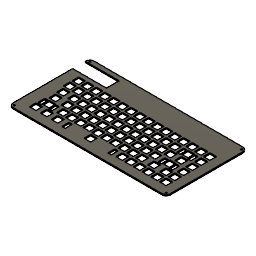
middle (Autodesk Fusion 360 design; units mm, degrees)
part number: 2026-05-16-15-46-12-709
Autodesk Fusion 360 part; units mm, degrees
(part 1 of 3)
sketch "Sketch1" plane through (0, 0, 0) normal (0, 0, 1) x (1, 0, 0)
  line L0 (228.9474, 57.4273) -> (228.9474, -118.8427)
  line L1 (-113.7226, 57.4273) -> (228.9474, 57.4273)
  line L2 (-113.7226, -118.8427) -> (-113.7226, 57.4273)
  line L3 (228.9474, -118.8427) -> (-113.7226, -118.8427)
  line L4 (-90.3928, 10.2823) -> (-77.3928, 10.2823)
  line L5 (-90.3928, -3.7177) -> (-77.3928, -3.7177)
  line L6 (-90.8928, 9.7823) -> (-90.8928, -3.2177)
  line L7 (-76.8928, 9.7823) -> (-76.8928, -3.2177)
  arc A0 (-90.3928, 10.2823) -> (-90.8928, 9.7823) centre (-90.3928, 9.7823) ccw
  arc A1 (-76.8928, 9.7823) -> (-77.3928, 10.2823) centre (-77.3928, 9.7823) ccw
  arc A2 (-90.8928, -3.2177) -> (-90.3928, -3.7177) centre (-90.3928, -3.2177) ccw
  arc A3 (-77.3928, -3.7177) -> (-76.8928, -3.2177) centre (-77.3928, -3.2177) ccw
  line L8 (-71.3428, 10.2823) -> (-58.3428, 10.2823)
  line L9 (-71.3428, -3.7177) -> (-58.3428, -3.7177)
  line L10 (-71.8428, 9.7823) -> (-71.8428, -3.2177)
  line L11 (-57.8428, 9.7823) -> (-57.8428, -3.2177)
  arc A4 (-71.3428, 10.2823) -> (-71.8428, 9.7823) centre (-71.3428, 9.7823) ccw
  arc A5 (-57.8428, 9.7823) -> (-58.3428, 10.2823) centre (-58.3428, 9.7823) ccw
  arc A6 (-71.8428, -3.2177) -> (-71.3428, -3.7177) centre (-71.3428, -3.2177) ccw
  arc A7 (-58.3428, -3.7177) -> (-57.8428, -3.2177) centre (-58.3428, -3.2177) ccw
  line L12 (-52.2928, 10.2823) -> (-39.2928, 10.2823)
  line L13 (-52.2928, -3.7177) -> (-39.2928, -3.7177)
  line L14 (-52.7928, 9.7823) -> (-52.7928, -3.2177)
  line L15 (-38.7928, 9.7823) -> (-38.7928, -3.2177)
  arc A8 (-52.2928, 10.2823) -> (-52.7928, 9.7823) centre (-52.2928, 9.7823) ccw
  arc A9 (-38.7928, 9.7823) -> (-39.2928, 10.2823) centre (-39.2928, 9.7823) ccw
  arc A10 (-52.7928, -3.2177) -> (-52.2928, -3.7177) centre (-52.2928, -3.2177) ccw
  arc A11 (-39.2928, -3.7177) -> (-38.7928, -3.2177) centre (-39.2928, -3.2177) ccw
  line L16 (-33.2428, 10.2823) -> (-20.2428, 10.2823)
  line L17 (-33.2428, -3.7177) -> (-20.2428, -3.7177)
  line L18 (-33.7428, 9.7823) -> (-33.7428, -3.2177)
  line L19 (-19.7428, 9.7823) -> (-19.7428, -3.2177)
  arc A12 (-33.2428, 10.2823) -> (-33.7428, 9.7823) centre (-33.2428, 9.7823) ccw
  arc A13 (-19.7428, 9.7823) -> (-20.2428, 10.2823) centre (-20.2428, 9.7823) ccw
  arc A14 (-33.7428, -3.2177) -> (-33.2428, -3.7177) centre (-33.2428, -3.2177) ccw
  arc A15 (-20.2428, -3.7177) -> (-19.7428, -3.2177) centre (-20.2428, -3.2177) ccw
  line L20 (-14.1928, 10.2823) -> (-1.1928, 10.2823)
  line L21 (-14.1928, -3.7177) -> (-1.1928, -3.7177)
  line L22 (-14.6928, 9.7823) -> (-14.6928, -3.2177)
  line L23 (-0.6928, 9.7823) -> (-0.6928, -3.2177)
  arc A16 (-14.1928, 10.2823) -> (-14.6928, 9.7823) centre (-14.1928, 9.7823) ccw
  arc A17 (-0.6928, 9.7823) -> (-1.1928, 10.2823) centre (-1.1928, 9.7823) ccw
  arc A18 (-14.6928, -3.2177) -> (-14.1928, -3.7177) centre (-14.1928, -3.2177) ccw
  arc A19 (-1.1928, -3.7177) -> (-0.6928, -3.2177) centre (-1.1928, -3.2177) ccw
  line L24 (4.8572, 10.2823) -> (17.8572, 10.2823)
  line L25 (4.8572, -3.7177) -> (17.8572, -3.7177)
  line L26 (4.3572, 9.7823) -> (4.3572, -3.2177)
  line L27 (18.3572, 9.7823) -> (18.3572, -3.2177)
  arc A20 (4.8572, 10.2823) -> (4.3572, 9.7823) centre (4.8572, 9.7823) ccw
  arc A21 (18.3572, 9.7823) -> (17.8572, 10.2823) centre (17.8572, 9.7823) ccw
  arc A22 (4.3572, -3.2177) -> (4.8572, -3.7177) centre (4.8572, -3.2177) ccw
  arc A23 (17.8572, -3.7177) -> (18.3572, -3.2177) centre (17.8572, -3.2177) ccw
  line L28 (23.9072, 10.2823) -> (36.9072, 10.2823)
  line L29 (23.9072, -3.7177) -> (36.9072, -3.7177)
  line L30 (23.4072, 9.7823) -> (23.4072, -3.2177)
  line L31 (37.4072, 9.7823) -> (37.4072, -3.2177)
  arc A24 (23.9072, 10.2823) -> (23.4072, 9.7823) centre (23.9072, 9.7823) ccw
  arc A25 (37.4072, 9.7823) -> (36.9072, 10.2823) centre (36.9072, 9.7823) ccw
  arc A26 (23.4072, -3.2177) -> (23.9072, -3.7177) centre (23.9072, -3.2177) ccw
  arc A27 (36.9072, -3.7177) -> (37.4072, -3.2177) centre (36.9072, -3.2177) ccw
  line L32 (42.9572, 10.2823) -> (55.9572, 10.2823)
  line L33 (42.9572, -3.7177) -> (55.9572, -3.7177)
  line L34 (42.4572, 9.7823) -> (42.4572, -3.2177)
  line L35 (56.4572, 9.7823) -> (56.4572, -3.2177)
  arc A28 (42.9572, 10.2823) -> (42.4572, 9.7823) centre (42.9572, 9.7823) ccw
  arc A29 (56.4572, 9.7823) -> (55.9572, 10.2823) centre (55.9572, 9.7823) ccw
  arc A30 (42.4572, -3.2177) -> (42.9572, -3.7177) centre (42.9572, -3.2177) ccw
  arc A31 (55.9572, -3.7177) -> (56.4572, -3.2177) centre (55.9572, -3.2177) ccw
  line L36 (62.0072, 10.2823) -> (75.0072, 10.2823)
  line L37 (62.0072, -3.7177) -> (75.0072, -3.7177)
  line L38 (61.5072, 9.7823) -> (61.5072, -3.2177)
  line L39 (75.5072, 9.7823) -> (75.5072, -3.2177)
  arc A32 (62.0072, 10.2823) -> (61.5072, 9.7823) centre (62.0072, 9.7823) ccw
  arc A33 (75.5072, 9.7823) -> (75.0072, 10.2823) centre (75.0072, 9.7823) ccw
  arc A34 (61.5072, -3.2177) -> (62.0072, -3.7177) centre (62.0072, -3.2177) ccw
  arc A35 (75.0072, -3.7177) -> (75.5072, -3.2177) centre (75.0072, -3.2177) ccw
  line L40 (81.0572, 10.2823) -> (94.0572, 10.2823)
  line L41 (81.0572, -3.7177) -> (94.0572, -3.7177)
  line L42 (80.5572, 9.7823) -> (80.5572, -3.2177)
  line L43 (94.5572, 9.7823) -> (94.5572, -3.2177)
  arc A36 (81.0572, 10.2823) -> (80.5572, 9.7823) centre (81.0572, 9.7823) ccw
  arc A37 (94.5572, 9.7823) -> (94.0572, 10.2823) centre (94.0572, 9.7823) ccw
  arc A38 (80.5572, -3.2177) -> (81.0572, -3.7177) centre (81.0572, -3.2177) ccw
  arc A39 (94.0572, -3.7177) -> (94.5572, -3.2177) centre (94.0572, -3.2177) ccw
  line L44 (100.1072, 10.2823) -> (113.1072, 10.2823)
  line L45 (100.1072, -3.7177) -> (113.1072, -3.7177)
  line L46 (99.6072, 9.7823) -> (99.6072, -3.2177)
  line L47 (113.6072, 9.7823) -> (113.6072, -3.2177)
  arc A40 (100.1072, 10.2823) -> (99.6072, 9.7823) centre (100.1072, 9.7823) ccw
  arc A41 (113.6072, 9.7823) -> (113.1072, 10.2823) centre (113.1072, 9.7823) ccw
  arc A42 (99.6072, -3.2177) -> (100.1072, -3.7177) centre (100.1072, -3.2177) ccw
  arc A43 (113.1072, -3.7177) -> (113.6072, -3.2177) centre (113.1072, -3.2177) ccw
  line L48 (119.1572, 10.2823) -> (132.1572, 10.2823)
  line L49 (119.1572, -3.7177) -> (132.1572, -3.7177)
  line L50 (118.6572, 9.7823) -> (118.6572, -3.2177)
  line L51 (132.6572, 9.7823) -> (132.6572, -3.2177)
  arc A44 (119.1572, 10.2823) -> (118.6572, 9.7823) centre (119.1572, 9.7823) ccw
  arc A45 (132.6572, 9.7823) -> (132.1572, 10.2823) centre (132.1572, 9.7823) ccw
  arc A46 (118.6572, -3.2177) -> (119.1572, -3.7177) centre (119.1572, -3.2177) ccw
  arc A47 (132.1572, -3.7177) -> (132.6572, -3.2177) centre (132.1572, -3.2177) ccw
  line L52 (138.2072, 10.2823) -> (151.2072, 10.2823)
  line L53 (138.2072, -3.7177) -> (151.2072, -3.7177)
  line L54 (137.7072, 9.7823) -> (137.7072, -3.2177)
  line L55 (151.7072, 9.7823) -> (151.7072, -3.2177)
  arc A48 (138.2072, 10.2823) -> (137.7072, 9.7823) centre (138.2072, 9.7823) ccw
  arc A49 (151.7072, 9.7823) -> (151.2072, 10.2823) centre (151.2072, 9.7823) ccw
  arc A50 (137.7072, -3.2177) -> (138.2072, -3.7177) centre (138.2072, -3.2177) ccw
  arc A51 (151.2072, -3.7177) -> (151.7072, -3.2177) centre (151.2072, -3.2177) ccw
  line L56 (157.2572, 10.2823) -> (170.2572, 10.2823)
  line L57 (157.2572, -3.7177) -> (170.2572, -3.7177)
  line L58 (156.7572, 9.7823) -> (156.7572, -3.2177)
  line L59 (170.7572, 9.7823) -> (170.7572, -3.2177)
  arc A52 (157.2572, 10.2823) -> (156.7572, 9.7823) centre (157.2572, 9.7823) ccw
  arc A53 (170.7572, 9.7823) -> (170.2572, 10.2823) centre (170.2572, 9.7823) ccw
  arc A54 (156.7572, -3.2177) -> (157.2572, -3.7177) centre (157.2572, -3.2177) ccw
  arc A55 (170.2572, -3.7177) -> (170.7572, -3.2177) centre (170.2572, -3.2177) ccw
  line L60 (176.3072, 10.2823) -> (189.3072, 10.2823)
  line L61 (176.3072, -3.7177) -> (189.3072, -3.7177)
  line L62 (175.8072, 9.7823) -> (175.8072, -3.2177)
  line L63 (189.8072, 9.7823) -> (189.8072, -3.2177)
  arc A56 (176.3072, 10.2823) -> (175.8072, 9.7823) centre (176.3072, 9.7823) ccw
  arc A57 (189.8072, 9.7823) -> (189.3072, 10.2823) centre (189.3072, 9.7823) ccw
  arc A58 (175.8072, -3.2177) -> (176.3072, -3.7177) centre (176.3072, -3.2177) ccw
  arc A59 (189.3072, -3.7177) -> (189.8072, -3.2177) centre (189.3072, -3.2177) ccw
  line L64 (195.3572, 10.2823) -> (208.3572, 10.2823)
  line L65 (195.3572, -3.7177) -> (208.3572, -3.7177)
  line L66 (194.8572, 9.7823) -> (194.8572, -3.2177)
  line L67 (208.8572, 9.7823) -> (208.8572, -3.2177)
  arc A60 (195.3572, 10.2823) -> (194.8572, 9.7823) centre (195.3572, 9.7823) ccw
  arc A61 (208.8572, 9.7823) -> (208.3572, 10.2823) centre (208.3572, 9.7823) ccw
  arc A62 (194.8572, -3.2177) -> (195.3572, -3.7177) centre (195.3572, -3.2177) ccw
  arc A63 (208.3572, -3.7177) -> (208.8572, -3.2177) centre (208.3572, -3.2177) ccw
  line L68 (-90.3928, -8.7677) -> (-77.3928, -8.7677)
  line L69 (-90.3928, -22.7677) -> (-77.3928, -22.7677)
  line L70 (-90.8928, -9.2677) -> (-90.8928, -22.2677)
  line L71 (-76.8928, -9.2677) -> (-76.8928, -22.2677)
  arc A64 (-90.3928, -8.7677) -> (-90.8928, -9.2677) centre (-90.3928, -9.2677) ccw
  arc A65 (-76.8928, -9.2677) -> (-77.3928, -8.7677) centre (-77.3928, -9.2677) ccw
  arc A66 (-90.8928, -22.2677) -> (-90.3928, -22.7677) centre (-90.3928, -22.2677) ccw
  arc A67 (-77.3928, -22.7677) -> (-76.8928, -22.2677) centre (-77.3928, -22.2677) ccw
  line L72 (-71.3428, -8.7677) -> (-58.3428, -8.7677)
  line L73 (-71.3428, -22.7677) -> (-58.3428, -22.7677)
  line L74 (-71.8428, -9.2677) -> (-71.8428, -22.2677)
  line L75 (-57.8428, -9.2677) -> (-57.8428, -22.2677)
  arc A68 (-71.3428, -8.7677) -> (-71.8428, -9.2677) centre (-71.3428, -9.2677) ccw
  arc A69 (-57.8428, -9.2677) -> (-58.3428, -8.7677) centre (-58.3428, -9.2677) ccw
  arc A70 (-71.8428, -22.2677) -> (-71.3428, -22.7677) centre (-71.3428, -22.2677) ccw
  arc A71 (-58.3428, -22.7677) -> (-57.8428, -22.2677) centre (-58.3428, -22.2677) ccw
  line L76 (-52.2928, -8.7677) -> (-39.2928, -8.7677)
  line L77 (-52.2928, -22.7677) -> (-39.2928, -22.7677)
  line L78 (-52.7928, -9.2677) -> (-52.7928, -22.2677)
  line L79 (-38.7928, -9.2677) -> (-38.7928, -22.2677)
  arc A72 (-52.2928, -8.7677) -> (-52.7928, -9.2677) centre (-52.2928, -9.2677) ccw
  arc A73 (-38.7928, -9.2677) -> (-39.2928, -8.7677) centre (-39.2928, -9.2677) ccw
  arc A74 (-52.7928, -22.2677) -> (-52.2928, -22.7677) centre (-52.2928, -22.2677) ccw
  arc A75 (-39.2928, -22.7677) -> (-38.7928, -22.2677) centre (-39.2928, -22.2677) ccw
  line L80 (-33.2428, -8.7677) -> (-20.2428, -8.7677)
  line L81 (-33.2428, -22.7677) -> (-20.2428, -22.7677)
  line L82 (-33.7428, -9.2677) -> (-33.7428, -22.2677)
  line L83 (-19.7428, -9.2677) -> (-19.7428, -22.2677)
  arc A76 (-33.2428, -8.7677) -> (-33.7428, -9.2677) centre (-33.2428, -9.2677) ccw
  arc A77 (-19.7428, -9.2677) -> (-20.2428, -8.7677) centre (-20.2428, -9.2677) ccw
  arc A78 (-33.7428, -22.2677) -> (-33.2428, -22.7677) centre (-33.2428, -22.2677) ccw
  arc A79 (-20.2428, -22.7677) -> (-19.7428, -22.2677) centre (-20.2428, -22.2677) ccw
  line L84 (-14.1928, -8.7677) -> (-1.1928, -8.7677)
  line L85 (-14.1928, -22.7677) -> (-1.1928, -22.7677)
  line L86 (-14.6928, -9.2677) -> (-14.6928, -22.2677)
  line L87 (-0.6928, -9.2677) -> (-0.6928, -22.2677)
  arc A80 (-14.1928, -8.7677) -> (-14.6928, -9.2677) centre (-14.1928, -9.2677) ccw
  arc A81 (-0.6928, -9.2677) -> (-1.1928, -8.7677) centre (-1.1928, -9.2677) ccw
  arc A82 (-14.6928, -22.2677) -> (-14.1928, -22.7677) centre (-14.1928, -22.2677) ccw
  arc A83 (-1.1928, -22.7677) -> (-0.6928, -22.2677) centre (-1.1928, -22.2677) ccw
  line L88 (4.8572, -8.7677) -> (17.8572, -8.7677)
  line L89 (4.8572, -22.7677) -> (17.8572, -22.7677)
  line L90 (4.3572, -9.2677) -> (4.3572, -22.2677)
  line L91 (18.3572, -9.2677) -> (18.3572, -22.2677)
  arc A84 (4.8572, -8.7677) -> (4.3572, -9.2677) centre (4.8572, -9.2677) ccw
  arc A85 (18.3572, -9.2677) -> (17.8572, -8.7677) centre (17.8572, -9.2677) ccw
  arc A86 (4.3572, -22.2677) -> (4.8572, -22.7677) centre (4.8572, -22.2677) ccw
  arc A87 (17.8572, -22.7677) -> (18.3572, -22.2677) centre (17.8572, -22.2677) ccw
  line L92 (23.9072, -8.7677) -> (36.9072, -8.7677)
  line L93 (23.9072, -22.7677) -> (36.9072, -22.7677)
  line L94 (23.4072, -9.2677) -> (23.4072, -22.2677)
  line L95 (37.4072, -9.2677) -> (37.4072, -22.2677)
  arc A88 (23.9072, -8.7677) -> (23.4072, -9.2677) centre (23.9072, -9.2677) ccw
  arc A89 (37.4072, -9.2677) -> (36.9072, -8.7677) centre (36.9072, -9.2677) ccw
  arc A90 (23.4072, -22.2677) -> (23.9072, -22.7677) centre (23.9072, -22.2677) ccw
  arc A91 (36.9072, -22.7677) -> (37.4072, -22.2677) centre (36.9072, -22.2677) ccw
  line L96 (42.9572, -8.7677) -> (55.9572, -8.7677)
  line L97 (42.9572, -22.7677) -> (55.9572, -22.7677)
  line L98 (42.4572, -9.2677) -> (42.4572, -22.2677)
  line L99 (56.4572, -9.2677) -> (56.4572, -22.2677)
  arc A92 (42.9572, -8.7677) -> (42.4572, -9.2677) centre (42.9572, -9.2677) ccw
  arc A93 (56.4572, -9.2677) -> (55.9572, -8.7677) centre (55.9572, -9.2677) ccw
  arc A94 (42.4572, -22.2677) -> (42.9572, -22.7677) centre (42.9572, -22.2677) ccw
  arc A95 (55.9572, -22.7677) -> (56.4572, -22.2677) centre (55.9572, -22.2677) ccw
  line L100 (62.0072, -8.7677) -> (75.0072, -8.7677)
  line L101 (62.0072, -22.7677) -> (75.0072, -22.7677)
  line L102 (61.5072, -9.2677) -> (61.5072, -22.2677)
  line L103 (75.5072, -9.2677) -> (75.5072, -22.2677)
  arc A96 (62.0072, -8.7677) -> (61.5072, -9.2677) centre (62.0072, -9.2677) ccw
  arc A97 (75.5072, -9.2677) -> (75.0072, -8.7677) centre (75.0072, -9.2677) ccw
  arc A98 (61.5072, -22.2677) -> (62.0072, -22.7677) centre (62.0072, -22.2677) ccw
  arc A99 (75.0072, -22.7677) -> (75.5072, -22.2677) centre (75.0072, -22.2677) ccw
  line L104 (81.0572, -8.7677) -> (94.0572, -8.7677)
  line L105 (81.0572, -22.7677) -> (94.0572, -22.7677)
  line L106 (80.5572, -9.2677) -> (80.5572, -22.2677)
  line L107 (94.5572, -9.2677) -> (94.5572, -22.2677)
  arc A100 (81.0572, -8.7677) -> (80.5572, -9.2677) centre (81.0572, -9.2677) ccw
  arc A101 (94.5572, -9.2677) -> (94.0572, -8.7677) centre (94.0572, -9.2677) ccw
  arc A102 (80.5572, -22.2677) -> (81.0572, -22.7677) centre (81.0572, -22.2677) ccw
  arc A103 (94.0572, -22.7677) -> (94.5572, -22.2677) centre (94.0572, -22.2677) ccw
  line L108 (100.1072, -8.7677) -> (113.1072, -8.7677)
  line L109 (100.1072, -22.7677) -> (113.1072, -22.7677)
  line L110 (99.6072, -9.2677) -> (99.6072, -22.2677)
  line L111 (113.6072, -9.2677) -> (113.6072, -22.2677)
  arc A104 (100.1072, -8.7677) -> (99.6072, -9.2677) centre (100.1072, -9.2677) ccw
  arc A105 (113.6072, -9.2677) -> (113.1072, -8.7677) centre (113.1072, -9.2677) ccw
  arc A106 (99.6072, -22.2677) -> (100.1072, -22.7677) centre (100.1072, -22.2677) ccw
  arc A107 (113.1072, -22.7677) -> (113.6072, -22.2677) centre (113.1072, -22.2677) ccw
  line L112 (119.1572, -8.7677) -> (132.1572, -8.7677)
  line L113 (119.1572, -22.7677) -> (132.1572, -22.7677)
  line L114 (118.6572, -9.2677) -> (118.6572, -22.2677)
  line L115 (132.6572, -9.2677) -> (132.6572, -22.2677)
  arc A108 (119.1572, -8.7677) -> (118.6572, -9.2677) centre (119.1572, -9.2677) ccw
  arc A109 (132.6572, -9.2677) -> (132.1572, -8.7677) centre (132.1572, -9.2677) ccw
  arc A110 (118.6572, -22.2677) -> (119.1572, -22.7677) centre (119.1572, -22.2677) ccw
  arc A111 (132.1572, -22.7677) -> (132.6572, -22.2677) centre (132.1572, -22.2677) ccw
  line L116 (138.2072, -8.7677) -> (151.2072, -8.7677)
  line L117 (138.2072, -22.7677) -> (151.2072, -22.7677)
  line L118 (137.7072, -9.2677) -> (137.7072, -22.2677)
  line L119 (151.7072, -9.2677) -> (151.7072, -22.2677)
  arc A112 (138.2072, -8.7677) -> (137.7072, -9.2677) centre (138.2072, -9.2677) ccw
  arc A113 (151.7072, -9.2677) -> (151.2072, -8.7677) centre (151.2072, -9.2677) ccw
  arc A114 (137.7072, -22.2677) -> (138.2072, -22.7677) centre (138.2072, -22.2677) ccw
  arc A115 (151.2072, -22.7677) -> (151.7072, -22.2677) centre (151.2072, -22.2677) ccw
  line L120 (166.7822, -8.7677) -> (179.7822, -8.7677)
  line L121 (166.7822, -22.7677) -> (179.7822, -22.7677)
  line L122 (166.2822, -9.2677) -> (166.2822, -22.2677)
  line L123 (180.2822, -9.2677) -> (180.2822, -22.2677)
  arc A116 (166.7822, -8.7677) -> (166.2822, -9.2677) centre (166.7822, -9.2677) ccw
  arc A117 (180.2822, -9.2677) -> (179.7822, -8.7677) centre (179.7822, -9.2677) ccw
  arc A118 (166.2822, -22.2677) -> (166.7822, -22.7677) centre (166.7822, -22.2677) ccw
  arc A119 (179.7822, -22.7677) -> (180.2822, -22.2677) centre (179.7822, -22.2677) ccw
  line L124 (158.3442, -9.7677) -> (164.3442, -9.7677)
  line L125 (158.3442, -24.7677) -> (164.3442, -24.7677)
  line L126 (157.8442, -10.2677) -> (157.8442, -24.2677)
  line L127 (164.8442, -10.2677) -> (164.8442, -24.2677)
  arc A120 (158.3442, -9.7677) -> (157.8442, -10.2677) centre (158.3442, -10.2677) ccw
  arc A121 (164.8442, -10.2677) -> (164.3442, -9.7677) centre (164.3442, -10.2677) ccw
  arc A122 (157.8442, -24.2677) -> (158.3442, -24.7677) centre (158.3442, -24.2677) ccw
  arc A123 (164.3442, -24.7677) -> (164.8442, -24.2677) centre (164.3442, -24.2677) ccw
  line L128 (182.2202, -9.7677) -> (188.2202, -9.7677)
  line L129 (182.2202, -24.7677) -> (188.2202, -24.7677)
  line L130 (181.7202, -10.2677) -> (181.7202, -24.2677)
  line L131 (188.7202, -10.2677) -> (188.7202, -24.2677)
  arc A124 (182.2202, -9.7677) -> (181.7202, -10.2677) centre (182.2202, -10.2677) ccw
  arc A125 (188.7202, -10.2677) -> (188.2202, -9.7677) centre (188.2202, -10.2677) ccw
  arc A126 (181.7202, -24.2677) -> (182.2202, -24.7677) centre (182.2202, -24.2677) ccw
  arc A127 (188.2202, -24.7677) -> (188.7202, -24.2677) centre (188.2202, -24.2677) ccw
  line L132 (195.3572, -8.7677) -> (208.3572, -8.7677)
  line L133 (195.3572, -22.7677) -> (208.3572, -22.7677)
  line L134 (194.8572, -9.2677) -> (194.8572, -22.2677)
  line L135 (208.8572, -9.2677) -> (208.8572, -22.2677)
  arc A128 (195.3572, -8.7677) -> (194.8572, -9.2677) centre (195.3572, -9.2677) ccw
  arc A129 (208.8572, -9.2677) -> (208.3572, -8.7677) centre (208.3572, -9.2677) ccw
  arc A130 (194.8572, -22.2677) -> (195.3572, -22.7677) centre (195.3572, -22.2677) ccw
  arc A131 (208.3572, -22.7677) -> (208.8572, -22.2677) centre (208.3572, -22.2677) ccw
  line L136 (-85.6303, -27.8177) -> (-72.6303, -27.8177)
  line L137 (-85.6303, -41.8177) -> (-72.6303, -41.8177)
  line L138 (-86.1303, -28.3177) -> (-86.1303, -41.3177)
  line L139 (-72.1303, -28.3177) -> (-72.1303, -41.3177)
  arc A132 (-85.6303, -27.8177) -> (-86.1303, -28.3177) centre (-85.6303, -28.3177) ccw
  arc A133 (-72.1303, -28.3177) -> (-72.6303, -27.8177) centre (-72.6303, -28.3177) ccw
  arc A134 (-86.1303, -41.3177) -> (-85.6303, -41.8177) centre (-85.6303, -41.3177) ccw
  arc A135 (-72.6303, -41.8177) -> (-72.1303, -41.3177) centre (-72.6303, -41.3177) ccw
  line L140 (-61.8178, -27.8177) -> (-48.8178, -27.8177)
  line L141 (-61.8178, -41.8177) -> (-48.8178, -41.8177)
  line L142 (-62.3178, -28.3177) -> (-62.3178, -41.3177)
  line L143 (-48.3178, -28.3177) -> (-48.3178, -41.3177)
  arc A136 (-61.8178, -27.8177) -> (-62.3178, -28.3177) centre (-61.8178, -28.3177) ccw
  arc A137 (-48.3178, -28.3177) -> (-48.8178, -27.8177) centre (-48.8178, -28.3177) ccw
  arc A138 (-62.3178, -41.3177) -> (-61.8178, -41.8177) centre (-61.8178, -41.3177) ccw
  arc A139 (-48.8178, -41.8177) -> (-48.3178, -41.3177) centre (-48.8178, -41.3177) ccw
  line L144 (-42.7678, -27.8177) -> (-29.7678, -27.8177)
  line L145 (-42.7678, -41.8177) -> (-29.7678, -41.8177)
  line L146 (-43.2678, -28.3177) -> (-43.2678, -41.3177)
  line L147 (-29.2678, -28.3177) -> (-29.2678, -41.3177)
  arc A140 (-42.7678, -27.8177) -> (-43.2678, -28.3177) centre (-42.7678, -28.3177) ccw
  arc A141 (-29.2678, -28.3177) -> (-29.7678, -27.8177) centre (-29.7678, -28.3177) ccw
  arc A142 (-43.2678, -41.3177) -> (-42.7678, -41.8177) centre (-42.7678, -41.3177) ccw
  arc A143 (-29.7678, -41.8177) -> (-29.2678, -41.3177) centre (-29.7678, -41.3177) ccw
  line L148 (-23.7178, -27.8177) -> (-10.7178, -27.8177)
  line L149 (-23.7178, -41.8177) -> (-10.7178, -41.8177)
  line L150 (-24.2178, -28.3177) -> (-24.2178, -41.3177)
  line L151 (-10.2178, -28.3177) -> (-10.2178, -41.3177)
  arc A144 (-23.7178, -27.8177) -> (-24.2178, -28.3177) centre (-23.7178, -28.3177) ccw
  arc A145 (-10.2178, -28.3177) -> (-10.7178, -27.8177) centre (-10.7178, -28.3177) ccw
  arc A146 (-24.2178, -41.3177) -> (-23.7178, -41.8177) centre (-23.7178, -41.3177) ccw
  arc A147 (-10.7178, -41.8177) -> (-10.2178, -41.3177) centre (-10.7178, -41.3177) ccw
  line L152 (-4.6678, -27.8177) -> (8.3322, -27.8177)
  line L153 (-4.6678, -41.8177) -> (8.3322, -41.8177)
  line L154 (-5.1678, -28.3177) -> (-5.1678, -41.3177)
  line L155 (8.8322, -28.3177) -> (8.8322, -41.3177)
  arc A148 (-4.6678, -27.8177) -> (-5.1678, -28.3177) centre (-4.6678, -28.3177) ccw
  arc A149 (8.8322, -28.3177) -> (8.3322, -27.8177) centre (8.3322, -28.3177) ccw
  arc A150 (-5.1678, -41.3177) -> (-4.6678, -41.8177) centre (-4.6678, -41.3177) ccw
  arc A151 (8.3322, -41.8177) -> (8.8322, -41.3177) centre (8.3322, -41.3177) ccw
  line L156 (14.3822, -27.8177) -> (27.3822, -27.8177)
  line L157 (14.3822, -41.8177) -> (27.3822, -41.8177)
  line L158 (13.8822, -28.3177) -> (13.8822, -41.3177)
  line L159 (27.8822, -28.3177) -> (27.8822, -41.3177)
  arc A152 (14.3822, -27.8177) -> (13.8822, -28.3177) centre (14.3822, -28.3177) ccw
  arc A153 (27.8822, -28.3177) -> (27.3822, -27.8177) centre (27.3822, -28.3177) ccw
  arc A154 (13.8822, -41.3177) -> (14.3822, -41.8177) centre (14.3822, -41.3177) ccw
  arc A155 (27.3822, -41.8177) -> (27.8822, -41.3177) centre (27.3822, -41.3177) ccw
  line L160 (33.4322, -27.8177) -> (46.4322, -27.8177)
  line L161 (33.4322, -41.8177) -> (46.4322, -41.8177)
  line L162 (32.9322, -28.3177) -> (32.9322, -41.3177)
  line L163 (46.9322, -28.3177) -> (46.9322, -41.3177)
  arc A156 (33.4322, -27.8177) -> (32.9322, -28.3177) centre (33.4322, -28.3177) ccw
  arc A157 (46.9322, -28.3177) -> (46.4322, -27.8177) centre (46.4322, -28.3177) ccw
  arc A158 (32.9322, -41.3177) -> (33.4322, -41.8177) centre (33.4322, -41.3177) ccw
  arc A159 (46.4322, -41.8177) -> (46.9322, -41.3177) centre (46.4322, -41.3177) ccw
  line L164 (52.4822, -27.8177) -> (65.4822, -27.8177)
  line L165 (52.4822, -41.8177) -> (65.4822, -41.8177)
  line L166 (51.9822, -28.3177) -> (51.9822, -41.3177)
  line L167 (65.9822, -28.3177) -> (65.9822, -41.3177)
  arc A160 (52.4822, -27.8177) -> (51.9822, -28.3177) centre (52.4822, -28.3177) ccw
  arc A161 (65.9822, -28.3177) -> (65.4822, -27.8177) centre (65.4822, -28.3177) ccw
  arc A162 (51.9822, -41.3177) -> (52.4822, -41.8177) centre (52.4822, -41.3177) ccw
  arc A163 (65.4822, -41.8177) -> (65.9822, -41.3177) centre (65.4822, -41.3177) ccw
  line L168 (71.5322, -27.8177) -> (84.5322, -27.8177)
  line L169 (71.5322, -41.8177) -> (84.5322, -41.8177)
  line L170 (71.0322, -28.3177) -> (71.0322, -41.3177)
  line L171 (85.0322, -28.3177) -> (85.0322, -41.3177)
  arc A164 (71.5322, -27.8177) -> (71.0322, -28.3177) centre (71.5322, -28.3177) ccw
  arc A165 (85.0322, -28.3177) -> (84.5322, -27.8177) centre (84.5322, -28.3177) ccw
  arc A166 (71.0322, -41.3177) -> (71.5322, -41.8177) centre (71.5322, -41.3177) ccw
  arc A167 (84.5322, -41.8177) -> (85.0322, -41.3177) centre (84.5322, -41.3177) ccw
  line L172 (90.5822, -27.8177) -> (103.5822, -27.8177)
  line L173 (90.5822, -41.8177) -> (103.5822, -41.8177)
  line L174 (90.0822, -28.3177) -> (90.0822, -41.3177)
  line L175 (104.0822, -28.3177) -> (104.0822, -41.3177)
  arc A168 (90.5822, -27.8177) -> (90.0822, -28.3177) centre (90.5822, -28.3177) ccw
  arc A169 (104.0822, -28.3177) -> (103.5822, -27.8177) centre (103.5822, -28.3177) ccw
  arc A170 (90.0822, -41.3177) -> (90.5822, -41.8177) centre (90.5822, -41.3177) ccw
  arc A171 (103.5822, -41.8177) -> (104.0822, -41.3177) centre (103.5822, -41.3177) ccw
  line L176 (109.6322, -27.8177) -> (122.6322, -27.8177)
  line L177 (109.6322, -41.8177) -> (122.6322, -41.8177)
  line L178 (109.1322, -28.3177) -> (109.1322, -41.3177)
  line L179 (123.1322, -28.3177) -> (123.1322, -41.3177)
  arc A172 (109.6322, -27.8177) -> (109.1322, -28.3177) centre (109.6322, -28.3177) ccw
  arc A173 (123.1322, -28.3177) -> (122.6322, -27.8177) centre (122.6322, -28.3177) ccw
  arc A174 (109.1322, -41.3177) -> (109.6322, -41.8177) centre (109.6322, -41.3177) ccw
  arc A175 (122.6322, -41.8177) -> (123.1322, -41.3177) centre (122.6322, -41.3177) ccw
  line L180 (128.6822, -27.8177) -> (141.6822, -27.8177)
  line L181 (128.6822, -41.8177) -> (141.6822, -41.8177)
  line L182 (128.1822, -28.3177) -> (128.1822, -41.3177)
  line L183 (142.1822, -28.3177) -> (142.1822, -41.3177)
  arc A176 (128.6822, -27.8177) -> (128.1822, -28.3177) centre (128.6822, -28.3177) ccw
  arc A177 (142.1822, -28.3177) -> (141.6822, -27.8177) centre (141.6822, -28.3177) ccw
  arc A178 (128.1822, -41.3177) -> (128.6822, -41.8177) centre (128.6822, -41.3177) ccw
  arc A179 (141.6822, -41.8177) -> (142.1822, -41.3177) centre (141.6822, -41.3177) ccw
  line L184 (147.7322, -27.8177) -> (160.7322, -27.8177)
  line L185 (147.7322, -41.8177) -> (160.7322, -41.8177)
  line L186 (147.2322, -28.3177) -> (147.2322, -41.3177)
  line L187 (161.2322, -28.3177) -> (161.2322, -41.3177)
  arc A180 (147.7322, -27.8177) -> (147.2322, -28.3177) centre (147.7322, -28.3177) ccw
  arc A181 (161.2322, -28.3177) -> (160.7322, -27.8177) centre (160.7322, -28.3177) ccw
  arc A182 (147.2322, -41.3177) -> (147.7322, -41.8177) centre (147.7322, -41.3177) ccw
  arc A183 (160.7322, -41.8177) -> (161.2322, -41.3177) centre (160.7322, -41.3177) ccw
  line L188 (171.5447, -27.8177) -> (184.5447, -27.8177)
  line L189 (171.5447, -41.8177) -> (184.5447, -41.8177)
  line L190 (171.0447, -28.3177) -> (171.0447, -41.3177)
  line L191 (185.0447, -28.3177) -> (185.0447, -41.3177)
  arc A184 (171.5447, -27.8177) -> (171.0447, -28.3177) centre (171.5447, -28.3177) ccw
  arc A185 (185.0447, -28.3177) -> (184.5447, -27.8177) centre (184.5447, -28.3177) ccw
  arc A186 (171.0447, -41.3177) -> (171.5447, -41.8177) centre (171.5447, -41.3177) ccw
  arc A187 (184.5447, -41.8177) -> (185.0447, -41.3177) centre (184.5447, -41.3177) ccw
  line L192 (195.3572, -27.8177) -> (208.3572, -27.8177)
  line L193 (195.3572, -41.8177) -> (208.3572, -41.8177)
  line L194 (194.8572, -28.3177) -> (194.8572, -41.3177)
  line L195 (208.8572, -28.3177) -> (208.8572, -41.3177)
  arc A188 (195.3572, -27.8177) -> (194.8572, -28.3177) centre (195.3572, -28.3177) ccw
  arc A189 (208.8572, -28.3177) -> (208.3572, -27.8177) centre (208.3572, -28.3177) ccw
  arc A190 (194.8572, -41.3177) -> (195.3572, -41.8177) centre (195.3572, -41.3177) ccw
  arc A191 (208.3572, -41.8177) -> (208.8572, -41.3177) centre (208.3572, -41.3177) ccw
  line L196 (-83.2491, -46.8677) -> (-70.2491, -46.8677)
  line L197 (-83.2491, -60.8677) -> (-70.2491, -60.8677)
  line L198 (-83.7491, -47.3677) -> (-83.7491, -60.3677)
  line L199 (-69.7491, -47.3677) -> (-69.7491, -60.3677)
  arc A192 (-83.2491, -46.8677) -> (-83.7491, -47.3677) centre (-83.2491, -47.3677) ccw
  arc A193 (-69.7491, -47.3677) -> (-70.2491, -46.8677) centre (-70.2491, -47.3677) ccw
  arc A194 (-83.7491, -60.3677) -> (-83.2491, -60.8677) centre (-83.2491, -60.3677) ccw
  arc A195 (-70.2491, -60.8677) -> (-69.7491, -60.3677) centre (-70.2491, -60.3677) ccw
  line L200 (-57.0553, -46.8677) -> (-44.0553, -46.8677)
  line L201 (-57.0553, -60.8677) -> (-44.0553, -60.8677)
  line L202 (-57.5553, -47.3677) -> (-57.5553, -60.3677)
  line L203 (-43.5553, -47.3677) -> (-43.5553, -60.3677)
  arc A196 (-57.0553, -46.8677) -> (-57.5553, -47.3677) centre (-57.0553, -47.3677) ccw
  arc A197 (-43.5553, -47.3677) -> (-44.0553, -46.8677) centre (-44.0553, -47.3677) ccw
  arc A198 (-57.5553, -60.3677) -> (-57.0553, -60.8677) centre (-57.0553, -60.3677) ccw
  arc A199 (-44.0553, -60.8677) -> (-43.5553, -60.3677) centre (-44.0553, -60.3677) ccw
  line L204 (-38.0053, -46.8677) -> (-25.0053, -46.8677)
  line L205 (-38.0053, -60.8677) -> (-25.0053, -60.8677)
  line L206 (-38.5053, -47.3677) -> (-38.5053, -60.3677)
  line L207 (-24.5053, -47.3677) -> (-24.5053, -60.3677)
  arc A200 (-38.0053, -46.8677) -> (-38.5053, -47.3677) centre (-38.0053, -47.3677) ccw
  arc A201 (-24.5053, -47.3677) -> (-25.0053, -46.8677) centre (-25.0053, -47.3677) ccw
  arc A202 (-38.5053, -60.3677) -> (-38.0053, -60.8677) centre (-38.0053, -60.3677) ccw
  arc A203 (-25.0053, -60.8677) -> (-24.5053, -60.3677) centre (-25.0053, -60.3677) ccw
  line L208 (-18.9553, -46.8677) -> (-5.9553, -46.8677)
  line L209 (-18.9553, -60.8677) -> (-5.9553, -60.8677)
  line L210 (-19.4553, -47.3677) -> (-19.4553, -60.3677)
  line L211 (-5.4553, -47.3677) -> (-5.4553, -60.3677)
  arc A204 (-18.9553, -46.8677) -> (-19.4553, -47.3677) centre (-18.9553, -47.3677) ccw
  arc A205 (-5.4553, -47.3677) -> (-5.9553, -46.8677) centre (-5.9553, -47.3677) ccw
  arc A206 (-19.4553, -60.3677) -> (-18.9553, -60.8677) centre (-18.9553, -60.3677) ccw
  arc A207 (-5.9553, -60.8677) -> (-5.4553, -60.3677) centre (-5.9553, -60.3677) ccw
  line L212 (0.0947, -46.8677) -> (13.0947, -46.8677)
  line L213 (0.0947, -60.8677) -> (13.0947, -60.8677)
  line L214 (-0.4053, -47.3677) -> (-0.4053, -60.3677)
  line L215 (13.5947, -47.3677) -> (13.5947, -60.3677)
  arc A208 (0.0947, -46.8677) -> (-0.4053, -47.3677) centre (0.0947, -47.3677) ccw
  arc A209 (13.5947, -47.3677) -> (13.0947, -46.8677) centre (13.0947, -47.3677) ccw
  arc A210 (-0.4053, -60.3677) -> (0.0947, -60.8677) centre (0.0947, -60.3677) ccw
  arc A211 (13.0947, -60.8677) -> (13.5947, -60.3677) centre (13.0947, -60.3677) ccw
  line L216 (19.1447, -46.8677) -> (32.1447, -46.8677)
  line L217 (19.1447, -60.8677) -> (32.1447, -60.8677)
  line L218 (18.6447, -47.3677) -> (18.6447, -60.3677)
  line L219 (32.6447, -47.3677) -> (32.6447, -60.3677)
  arc A212 (19.1447, -46.8677) -> (18.6447, -47.3677) centre (19.1447, -47.3677) ccw
  arc A213 (32.6447, -47.3677) -> (32.1447, -46.8677) centre (32.1447, -47.3677) ccw
  arc A214 (18.6447, -60.3677) -> (19.1447, -60.8677) centre (19.1447, -60.3677) ccw
  arc A215 (32.1447, -60.8677) -> (32.6447, -60.3677) centre (32.1447, -60.3677) ccw
  line L220 (38.1947, -46.8677) -> (51.1947, -46.8677)
  line L221 (38.1947, -60.8677) -> (51.1947, -60.8677)
  line L222 (37.6947, -47.3677) -> (37.6947, -60.3677)
  line L223 (51.6947, -47.3677) -> (51.6947, -60.3677)
  arc A216 (38.1947, -46.8677) -> (37.6947, -47.3677) centre (38.1947, -47.3677) ccw
  arc A217 (51.6947, -47.3677) -> (51.1947, -46.8677) centre (51.1947, -47.3677) ccw
  arc A218 (37.6947, -60.3677) -> (38.1947, -60.8677) centre (38.1947, -60.3677) ccw
  arc A219 (51.1947, -60.8677) -> (51.6947, -60.3677) centre (51.1947, -60.3677) ccw
  line L224 (57.2447, -46.8677) -> (70.2447, -46.8677)
  line L225 (57.2447, -60.8677) -> (70.2447, -60.8677)
  line L226 (56.7447, -47.3677) -> (56.7447, -60.3677)
  line L227 (70.7447, -47.3677) -> (70.7447, -60.3677)
  arc A220 (57.2447, -46.8677) -> (56.7447, -47.3677) centre (57.2447, -47.3677) ccw
  arc A221 (70.7447, -47.3677) -> (70.2447, -46.8677) centre (70.2447, -47.3677) ccw
  arc A222 (56.7447, -60.3677) -> (57.2447, -60.8677) centre (57.2447, -60.3677) ccw
  arc A223 (70.2447, -60.8677) -> (70.7447, -60.3677) centre (70.2447, -60.3677) ccw
  line L228 (76.2947, -46.8677) -> (89.2947, -46.8677)
  line L229 (76.2947, -60.8677) -> (89.2947, -60.8677)
  line L230 (75.7947, -47.3677) -> (75.7947, -60.3677)
  line L231 (89.7947, -47.3677) -> (89.7947, -60.3677)
  arc A224 (76.2947, -46.8677) -> (75.7947, -47.3677) centre (76.2947, -47.3677) ccw
  arc A225 (89.7947, -47.3677) -> (89.2947, -46.8677) centre (89.2947, -47.3677) ccw
  arc A226 (75.7947, -60.3677) -> (76.2947, -60.8677) centre (76.2947, -60.3677) ccw
  arc A227 (89.2947, -60.8677) -> (89.7947, -60.3677) centre (89.2947, -60.3677) ccw
  line L232 (95.3447, -46.8677) -> (108.3447, -46.8677)
  line L233 (95.3447, -60.8677) -> (108.3447, -60.8677)
  line L234 (94.8447, -47.3677) -> (94.8447, -60.3677)
  line L235 (108.8447, -47.3677) -> (108.8447, -60.3677)
  arc A228 (95.3447, -46.8677) -> (94.8447, -47.3677) centre (95.3447, -47.3677) ccw
  arc A229 (108.8447, -47.3677) -> (108.3447, -46.8677) centre (108.3447, -47.3677) ccw
  arc A230 (94.8447, -60.3677) -> (95.3447, -60.8677) centre (95.3447, -60.3677) ccw
  arc A231 (108.3447, -60.8677) -> (108.8447, -60.3677) centre (108.3447, -60.3677) ccw
  line L236 (114.3947, -46.8677) -> (127.3947, -46.8677)
  line L237 (114.3947, -60.8677) -> (127.3947, -60.8677)
  line L238 (113.8947, -47.3677) -> (113.8947, -60.3677)
  line L239 (127.8947, -47.3677) -> (127.8947, -60.3677)
  arc A232 (114.3947, -46.8677) -> (113.8947, -47.3677) centre (114.3947, -47.3677) ccw
  arc A233 (127.8947, -47.3677) -> (127.3947, -46.8677) centre (127.3947, -47.3677) ccw
  arc A234 (113.8947, -60.3677) -> (114.3947, -60.8677) centre (114.3947, -60.3677) ccw
  arc A235 (127.3947, -60.8677) -> (127.8947, -60.3677) centre (127.3947, -60.3677) ccw
  line L240 (133.4447, -46.8677) -> (146.4447, -46.8677)
  line L241 (133.4447, -60.8677) -> (146.4447, -60.8677)
  line L242 (132.9447, -47.3677) -> (132.9447, -60.3677)
  line L243 (146.9447, -47.3677) -> (146.9447, -60.3677)
  arc A236 (133.4447, -46.8677) -> (132.9447, -47.3677) centre (133.4447, -47.3677) ccw
  arc A237 (146.9447, -47.3677) -> (146.4447, -46.8677) centre (146.4447, -47.3677) ccw
  arc A238 (132.9447, -60.3677) -> (133.4447, -60.8677) centre (133.4447, -60.3677) ccw
  arc A239 (146.4447, -60.8677) -> (146.9447, -60.3677) centre (146.4447, -60.3677) ccw
  line L244 (164.4009, -46.8677) -> (177.4009, -46.8677)
  line L245 (164.4009, -60.8677) -> (177.4009, -60.8677)
  line L246 (163.9009, -47.3677) -> (163.9009, -60.3677)
  line L247 (177.9009, -47.3677) -> (177.9009, -60.3677)
  arc A240 (164.4009, -46.8677) -> (163.9009, -47.3677) centre (164.4009, -47.3677) ccw
  arc A241 (177.9009, -47.3677) -> (177.4009, -46.8677) centre (177.4009, -47.3677) ccw
  arc A242 (163.9009, -60.3677) -> (164.4009, -60.8677) centre (164.4009, -60.3677) ccw
  arc A243 (177.4009, -60.8677) -> (177.9009, -60.3677) centre (177.4009, -60.3677) ccw
  line L248 (155.9629, -47.8677) -> (161.9629, -47.8677)
  line L249 (155.9629, -62.8677) -> (161.9629, -62.8677)
  line L250 (155.4629, -48.3677) -> (155.4629, -62.3677)
  line L251 (162.4629, -48.3677) -> (162.4629, -62.3677)
  arc A244 (155.9629, -47.8677) -> (155.4629, -48.3677) centre (155.9629, -48.3677) ccw
  arc A245 (162.4629, -48.3677) -> (161.9629, -47.8677) centre (161.9629, -48.3677) ccw
  arc A246 (155.4629, -62.3677) -> (155.9629, -62.8677) centre (155.9629, -62.3677) ccw
  arc A247 (161.9629, -62.8677) -> (162.4629, -62.3677) centre (161.9629, -62.3677) ccw
  line L252 (179.8389, -47.8677) -> (185.8389, -47.8677)
  line L253 (179.8389, -62.8677) -> (185.8389, -62.8677)
  line L254 (179.3389, -48.3677) -> (179.3389, -62.3677)
  line L255 (186.3389, -48.3677) -> (186.3389, -62.3677)
  arc A248 (179.8389, -47.8677) -> (179.3389, -48.3677) centre (179.8389, -48.3677) ccw
  arc A249 (186.3389, -48.3677) -> (185.8389, -47.8677) centre (185.8389, -48.3677) ccw
  arc A250 (179.3389, -62.3677) -> (179.8389, -62.8677) centre (179.8389, -62.3677) ccw
  arc A251 (185.8389, -62.8677) -> (186.3389, -62.3677) centre (185.8389, -62.3677) ccw
  line L256 (195.3572, -46.8677) -> (208.3572, -46.8677)
  line L257 (195.3572, -60.8677) -> (208.3572, -60.8677)
  line L258 (194.8572, -47.3677) -> (194.8572, -60.3677)
  line L259 (208.8572, -47.3677) -> (208.8572, -60.3677)
  arc A252 (195.3572, -46.8677) -> (194.8572, -47.3677) centre (195.3572, -47.3677) ccw
  arc A253 (208.8572, -47.3677) -> (208.3572, -46.8677) centre (208.3572, -47.3677) ccw
  arc A254 (194.8572, -60.3677) -> (195.3572, -60.8677) centre (195.3572, -60.3677) ccw
  arc A255 (208.3572, -60.8677) -> (208.8572, -60.3677) centre (208.3572, -60.3677) ccw
  line L260 (-78.4866, -65.9177) -> (-65.4866, -65.9177)
  line L261 (-78.4866, -79.9177) -> (-65.4866, -79.9177)
  line L262 (-78.9866, -66.4177) -> (-78.9866, -79.4177)
  line L263 (-64.9866, -66.4177) -> (-64.9866, -79.4177)
  arc A256 (-78.4866, -65.9177) -> (-78.9866, -66.4177) centre (-78.4866, -66.4177) ccw
  arc A257 (-64.9866, -66.4177) -> (-65.4866, -65.9177) centre (-65.4866, -66.4177) ccw
  arc A258 (-78.9866, -79.4177) -> (-78.4866, -79.9177) centre (-78.4866, -79.4177) ccw
  arc A259 (-65.4866, -79.9177) -> (-64.9866, -79.4177) centre (-65.4866, -79.4177) ccw
  line L264 (-86.9246, -66.9177) -> (-80.9246, -66.9177)
  line L265 (-86.9246, -81.9177) -> (-80.9246, -81.9177)
  line L266 (-87.4246, -67.4177) -> (-87.4246, -81.4177)
  line L267 (-80.4246, -67.4177) -> (-80.4246, -81.4177)
  arc A260 (-86.9246, -66.9177) -> (-87.4246, -67.4177) centre (-86.9246, -67.4177) ccw
  arc A261 (-80.4246, -67.4177) -> (-80.9246, -66.9177) centre (-80.9246, -67.4177) ccw
  arc A262 (-87.4246, -81.4177) -> (-86.9246, -81.9177) centre (-86.9246, -81.4177) ccw
  arc A263 (-80.9246, -81.9177) -> (-80.4246, -81.4177) centre (-80.9246, -81.4177) ccw
  line L268 (-63.0486, -66.9177) -> (-57.0486, -66.9177)
  line L269 (-63.0486, -81.9177) -> (-57.0486, -81.9177)
  line L270 (-63.5486, -67.4177) -> (-63.5486, -81.4177)
  line L271 (-56.5486, -67.4177) -> (-56.5486, -81.4177)
  arc A264 (-63.0486, -66.9177) -> (-63.5486, -67.4177) centre (-63.0486, -67.4177) ccw
  arc A265 (-56.5486, -67.4177) -> (-57.0486, -66.9177) centre (-57.0486, -67.4177) ccw
  arc A266 (-63.5486, -81.4177) -> (-63.0486, -81.9177) centre (-63.0486, -81.4177) ccw
  arc A267 (-57.0486, -81.9177) -> (-56.5486, -81.4177) centre (-57.0486, -81.4177) ccw
  line L272 (-47.5303, -65.9177) -> (-34.5303, -65.9177)
  line L273 (-47.5303, -79.9177) -> (-34.5303, -79.9177)
  line L274 (-48.0303, -66.4177) -> (-48.0303, -79.4177)
  line L275 (-34.0303, -66.4177) -> (-34.0303, -79.4177)
  arc A268 (-47.5303, -65.9177) -> (-48.0303, -66.4177) centre (-47.5303, -66.4177) ccw
  arc A269 (-34.0303, -66.4177) -> (-34.5303, -65.9177) centre (-34.5303, -66.4177) ccw
  arc A270 (-48.0303, -79.4177) -> (-47.5303, -79.9177) centre (-47.5303, -79.4177) ccw
  arc A271 (-34.5303, -79.9177) -> (-34.0303, -79.4177) centre (-34.5303, -79.4177) ccw
  line L276 (-28.4803, -65.9177) -> (-15.4803, -65.9177)
  line L277 (-28.4803, -79.9177) -> (-15.4803, -79.9177)
  line L278 (-28.9803, -66.4177) -> (-28.9803, -79.4177)
  line L279 (-14.9803, -66.4177) -> (-14.9803, -79.4177)
  arc A272 (-28.4803, -65.9177) -> (-28.9803, -66.4177) centre (-28.4803, -66.4177) ccw
  arc A273 (-14.9803, -66.4177) -> (-15.4803, -65.9177) centre (-15.4803, -66.4177) ccw
  arc A274 (-28.9803, -79.4177) -> (-28.4803, -79.9177) centre (-28.4803, -79.4177) ccw
  arc A275 (-15.4803, -79.9177) -> (-14.9803, -79.4177) centre (-15.4803, -79.4177) ccw
  line L280 (-9.4303, -65.9177) -> (3.5697, -65.9177)
  line L281 (-9.4303, -79.9177) -> (3.5697, -79.9177)
  line L282 (-9.9303, -66.4177) -> (-9.9303, -79.4177)
  line L283 (4.0697, -66.4177) -> (4.0697, -79.4177)
  arc A276 (-9.4303, -65.9177) -> (-9.9303, -66.4177) centre (-9.4303, -66.4177) ccw
  arc A277 (4.0697, -66.4177) -> (3.5697, -65.9177) centre (3.5697, -66.4177) ccw
  arc A278 (-9.9303, -79.4177) -> (-9.4303, -79.9177) centre (-9.4303, -79.4177) ccw
  arc A279 (3.5697, -79.9177) -> (4.0697, -79.4177) centre (3.5697, -79.4177) ccw
  line L284 (9.6197, -65.9177) -> (22.6197, -65.9177)
  line L285 (9.6197, -79.9177) -> (22.6197, -79.9177)
  line L286 (9.1197, -66.4177) -> (9.1197, -79.4177)
  line L287 (23.1197, -66.4177) -> (23.1197, -79.4177)
  arc A280 (9.6197, -65.9177) -> (9.1197, -66.4177) centre (9.6197, -66.4177) ccw
  arc A281 (23.1197, -66.4177) -> (22.6197, -65.9177) centre (22.6197, -66.4177) ccw
  arc A282 (9.1197, -79.4177) -> (9.6197, -79.9177) centre (9.6197, -79.4177) ccw
  arc A283 (22.6197, -79.9177) -> (23.1197, -79.4177) centre (22.6197, -79.4177) ccw
  line L288 (28.6697, -65.9177) -> (41.6697, -65.9177)
  line L289 (28.6697, -79.9177) -> (41.6697, -79.9177)
  line L290 (28.1697, -66.4177) -> (28.1697, -79.4177)
  line L291 (42.1697, -66.4177) -> (42.1697, -79.4177)
  arc A284 (28.6697, -65.9177) -> (28.1697, -66.4177) centre (28.6697, -66.4177) ccw
  arc A285 (42.1697, -66.4177) -> (41.6697, -65.9177) centre (41.6697, -66.4177) ccw
  arc A286 (28.1697, -79.4177) -> (28.6697, -79.9177) centre (28.6697, -79.4177) ccw
  arc A287 (41.6697, -79.9177) -> (42.1697, -79.4177) centre (41.6697, -79.4177) ccw
  line L292 (47.7197, -65.9177) -> (60.7197, -65.9177)
  line L293 (47.7197, -79.9177) -> (60.7197, -79.9177)
  line L294 (47.2197, -66.4177) -> (47.2197, -79.4177)
  line L295 (61.2197, -66.4177) -> (61.2197, -79.4177)
  arc A288 (47.7197, -65.9177) -> (47.2197, -66.4177) centre (47.7197, -66.4177) ccw
  arc A289 (61.2197, -66.4177) -> (60.7197, -65.9177) centre (60.7197, -66.4177) ccw
  arc A290 (47.2197, -79.4177) -> (47.7197, -79.9177) centre (47.7197, -79.4177) ccw
  arc A291 (60.7197, -79.9177) -> (61.2197, -79.4177) centre (60.7197, -79.4177) ccw
  line L296 (66.7697, -65.9177) -> (79.7697, -65.9177)
  line L297 (66.7697, -79.9177) -> (79.7697, -79.9177)
  line L298 (66.2697, -66.4177) -> (66.2697, -79.4177)
  line L299 (80.2697, -66.4177) -> (80.2697, -79.4177)
  arc A292 (66.7697, -65.9177) -> (66.2697, -66.4177) centre (66.7697, -66.4177) ccw
  arc A293 (80.2697, -66.4177) -> (79.7697, -65.9177) centre (79.7697, -66.4177) ccw
  arc A294 (66.2697, -79.4177) -> (66.7697, -79.9177) centre (66.7697, -79.4177) ccw
  arc A295 (79.7697, -79.9177) -> (80.2697, -79.4177) centre (79.7697, -79.4177) ccw
  line L300 (85.8197, -65.9177) -> (98.8197, -65.9177)
  line L301 (85.8197, -79.9177) -> (98.8197, -79.9177)
  line L302 (85.3197, -66.4177) -> (85.3197, -79.4177)
  line L303 (99.3197, -66.4177) -> (99.3197, -79.4177)
  arc A296 (85.8197, -65.9177) -> (85.3197, -66.4177) centre (85.8197, -66.4177) ccw
  arc A297 (99.3197, -66.4177) -> (98.8197, -65.9177) centre (98.8197, -66.4177) ccw
  arc A298 (85.3197, -79.4177) -> (85.8197, -79.9177) centre (85.8197, -79.4177) ccw
  arc A299 (98.8197, -79.9177) -> (99.3197, -79.4177) centre (98.8197, -79.4177) ccw
  line L304 (104.8697, -65.9177) -> (117.8697, -65.9177)
  line L305 (104.8697, -79.9177) -> (117.8697, -79.9177)
  line L306 (104.3697, -66.4177) -> (104.3697, -79.4177)
  line L307 (118.3697, -66.4177) -> (118.3697, -79.4177)
  arc A300 (104.8697, -65.9177) -> (104.3697, -66.4177) centre (104.8697, -66.4177) ccw
  arc A301 (118.3697, -66.4177) -> (117.8697, -65.9177) centre (117.8697, -66.4177) ccw
  arc A302 (104.3697, -79.4177) -> (104.8697, -79.9177) centre (104.8697, -79.4177) ccw
  arc A303 (117.8697, -79.9177) -> (118.3697, -79.4177) centre (117.8697, -79.4177) ccw
  line L308 (123.9197, -65.9177) -> (136.9197, -65.9177)
  line L309 (123.9197, -79.9177) -> (136.9197, -79.9177)
  line L310 (123.4197, -66.4177) -> (123.4197, -79.4177)
  line L311 (137.4197, -66.4177) -> (137.4197, -79.4177)
  arc A304 (123.9197, -65.9177) -> (123.4197, -66.4177) centre (123.9197, -66.4177) ccw
  arc A305 (137.4197, -66.4177) -> (136.9197, -65.9177) centre (136.9197, -66.4177) ccw
  arc A306 (123.4197, -79.4177) -> (123.9197, -79.9177) centre (123.9197, -79.4177) ccw
  arc A307 (136.9197, -79.9177) -> (137.4197, -79.4177) centre (136.9197, -79.4177) ccw
  line L312 (150.1134, -65.9177) -> (163.1134, -65.9177)
  line L313 (150.1134, -79.9177) -> (163.1134, -79.9177)
  line L314 (149.6134, -66.4177) -> (149.6134, -79.4177)
  line L315 (163.6134, -66.4177) -> (163.6134, -79.4177)
  arc A308 (150.1134, -65.9177) -> (149.6134, -66.4177) centre (150.1134, -66.4177) ccw
  arc A309 (163.6134, -66.4177) -> (163.1134, -65.9177) centre (163.1134, -66.4177) ccw
  arc A310 (149.6134, -79.4177) -> (150.1134, -79.9177) centre (150.1134, -79.4177) ccw
  arc A311 (163.1134, -79.9177) -> (163.6134, -79.4177) centre (163.1134, -79.4177) ccw
  line L316 (176.3072, -65.9177) -> (189.3072, -65.9177)
  line L317 (176.3072, -79.9177) -> (189.3072, -79.9177)
  line L318 (175.8072, -66.4177) -> (175.8072, -79.4177)
  line L319 (189.8072, -66.4177) -> (189.8072, -79.4177)
  arc A312 (176.3072, -65.9177) -> (175.8072, -66.4177) centre (176.3072, -66.4177) ccw
  arc A313 (189.8072, -66.4177) -> (189.3072, -65.9177) centre (189.3072, -66.4177) ccw
  arc A314 (175.8072, -79.4177) -> (176.3072, -79.9177) centre (176.3072, -79.4177) ccw
  arc A315 (189.3072, -79.9177) -> (189.8072, -79.4177) centre (189.3072, -79.4177) ccw
  line L320 (195.3572, -65.9177) -> (208.3572, -65.9177)
  line L321 (195.3572, -79.9177) -> (208.3572, -79.9177)
  line L322 (194.8572, -66.4177) -> (194.8572, -79.4177)
  line L323 (208.8572, -66.4177) -> (208.8572, -79.4177)
  arc A316 (195.3572, -65.9177) -> (194.8572, -66.4177) centre (195.3572, -66.4177) ccw
  arc A317 (208.8572, -66.4177) -> (208.3572, -65.9177) centre (208.3572, -66.4177) ccw
  arc A318 (194.8572, -79.4177) -> (195.3572, -79.9177) centre (195.3572, -79.4177) ccw
  arc A319 (208.3572, -79.9177) -> (208.8572, -79.4177) centre (208.3572, -79.4177) ccw
  line L324 (-88.0116, -84.9677) -> (-75.0116, -84.9677)
  line L325 (-88.0116, -98.9677) -> (-75.0116, -98.9677)
  line L326 (-88.5116, -85.4677) -> (-88.5116, -98.4677)
  line L327 (-74.5116, -85.4677) -> (-74.5116, -98.4677)
  arc A320 (-88.0116, -84.9677) -> (-88.5116, -85.4677) centre (-88.0116, -85.4677) ccw
  arc A321 (-74.5116, -85.4677) -> (-75.0116, -84.9677) centre (-75.0116, -85.4677) ccw
  arc A322 (-88.5116, -98.4677) -> (-88.0116, -98.9677) centre (-88.0116, -98.4677) ccw
  arc A323 (-75.0116, -98.9677) -> (-74.5116, -98.4677) centre (-75.0116, -98.4677) ccw
  line L328 (-64.1991, -84.9677) -> (-51.1991, -84.9677)
  line L329 (-64.1991, -98.9677) -> (-51.1991, -98.9677)
  line L330 (-64.6991, -85.4677) -> (-64.6991, -98.4677)
  line L331 (-50.6991, -85.4677) -> (-50.6991, -98.4677)
  arc A324 (-64.1991, -84.9677) -> (-64.6991, -85.4677) centre (-64.1991, -85.4677) ccw
  arc A325 (-50.6991, -85.4677) -> (-51.1991, -84.9677) centre (-51.1991, -85.4677) ccw
  arc A326 (-64.6991, -98.4677) -> (-64.1991, -98.9677) centre (-64.1991, -98.4677) ccw
  arc A327 (-51.1991, -98.9677) -> (-50.6991, -98.4677) centre (-51.1991, -98.4677) ccw
  line L332 (-40.3866, -84.9677) -> (-27.3866, -84.9677)
  line L333 (-40.3866, -98.9677) -> (-27.3866, -98.9677)
  line L334 (-40.8866, -85.4677) -> (-40.8866, -98.4677)
  line L335 (-26.8866, -85.4677) -> (-26.8866, -98.4677)
  arc A328 (-40.3866, -84.9677) -> (-40.8866, -85.4677) centre (-40.3866, -85.4677) ccw
  arc A329 (-26.8866, -85.4677) -> (-27.3866, -84.9677) centre (-27.3866, -85.4677) ccw
  arc A330 (-40.8866, -98.4677) -> (-40.3866, -98.9677) centre (-40.3866, -98.4677) ccw
  arc A331 (-27.3866, -98.9677) -> (-26.8866, -98.4677) centre (-27.3866, -98.4677) ccw
  line L336 (31.0509, -84.9677) -> (44.0509, -84.9677)
  line L337 (31.0509, -98.9677) -> (44.0509, -98.9677)
  line L338 (30.5509, -85.4677) -> (30.5509, -98.4677)
  line L339 (44.5509, -85.4677) -> (44.5509, -98.4677)
  arc A332 (31.0509, -84.9677) -> (30.5509, -85.4677) centre (31.0509, -85.4677) ccw
  arc A333 (44.5509, -85.4677) -> (44.0509, -84.9677) centre (44.0509, -85.4677) ccw
  arc A334 (30.5509, -98.4677) -> (31.0509, -98.9677) centre (31.0509, -98.4677) ccw
  arc A335 (44.0509, -98.9677) -> (44.5509, -98.4677) centre (44.0509, -98.4677) ccw
  line L340 (-15.4491, -85.9677) -> (-9.4491, -85.9677)
  line L341 (-15.4491, -100.9677) -> (-9.4491, -100.9677)
  line L342 (-15.9491, -86.4677) -> (-15.9491, -100.4677)
  line L343 (-8.9491, -86.4677) -> (-8.9491, -100.4677)
  arc A336 (-15.4491, -85.9677) -> (-15.9491, -86.4677) centre (-15.4491, -86.4677) ccw
  arc A337 (-8.9491, -86.4677) -> (-9.4491, -85.9677) centre (-9.4491, -86.4677) ccw
  arc A338 (-15.9491, -100.4677) -> (-15.4491, -100.9677) centre (-15.4491, -100.4677) ccw
  arc A339 (-9.4491, -100.9677) -> (-8.9491, -100.4677) centre (-9.4491, -100.4677) ccw
  line L344 (84.5509, -85.9677) -> (90.5509, -85.9677)
  line L345 (84.5509, -100.9677) -> (90.5509, -100.9677)
  line L346 (84.0509, -86.4677) -> (84.0509, -100.4677)
  line L347 (91.0509, -86.4677) -> (91.0509, -100.4677)
  arc A340 (84.5509, -85.9677) -> (84.0509, -86.4677) centre (84.5509, -86.4677) ccw
  arc A341 (91.0509, -86.4677) -> (90.5509, -85.9677) centre (90.5509, -86.4677) ccw
  arc A342 (84.0509, -100.4677) -> (84.5509, -100.9677) centre (84.5509, -100.4677) ccw
  arc A343 (90.5509, -100.9677) -> (91.0509, -100.4677) centre (90.5509, -100.4677) ccw
  line L348 (100.1072, -84.9677) -> (113.1072, -84.9677)
  line L349 (100.1072, -98.9677) -> (113.1072, -98.9677)
  line L350 (99.6072, -85.4677) -> (99.6072, -98.4677)
  line L351 (113.6072, -85.4677) -> (113.6072, -98.4677)
  arc A344 (100.1072, -84.9677) -> (99.6072, -85.4677) centre (100.1072, -85.4677) ccw
  arc A345 (113.6072, -85.4677) -> (113.1072, -84.9677) centre (113.1072, -85.4677) ccw
  arc A346 (99.6072, -98.4677) -> (100.1072, -98.9677) centre (100.1072, -98.4677) ccw
  arc A347 (113.1072, -98.9677) -> (113.6072, -98.4677) centre (113.1072, -98.4677) ccw
  line L352 (119.1572, -84.9677) -> (132.1572, -84.9677)
  line L353 (119.1572, -98.9677) -> (132.1572, -98.9677)
  line L354 (118.6572, -85.4677) -> (118.6572, -98.4677)
  line L355 (132.6572, -85.4677) -> (132.6572, -98.4677)
  arc A348 (119.1572, -84.9677) -> (118.6572, -85.4677) centre (119.1572, -85.4677) ccw
  arc A349 (132.6572, -85.4677) -> (132.1572, -84.9677) centre (132.1572, -85.4677) ccw